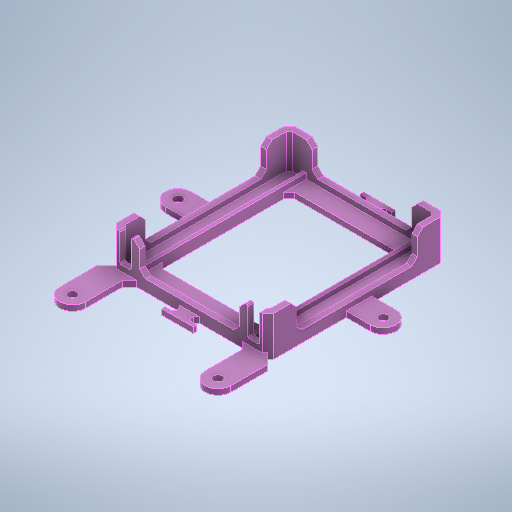
# Autodesk Inventor part: Battery-Holder-SPG27-1x4-A
Saved by Autodesk Inventor 2025.3 (Build 293356000, 356)
## iProperties
Created: 2025-09-09
Part Number: Battery-Holder-SPG27-1x4-A
Material: 一般
Document SubType Name: Modeling
Designer: daisuke
Density: 1 g/cm^3
Appearance: 滑らか - 紫
Author: daisuke
Autodesk Inventor part; units mm, degrees
ref_plane "YZ Plane" through (0, 0, 0) normal (1, 0, 0) x (0, 1, 0)
ref_plane "XZ Plane" through (0, 0, 0) normal (0, 1, 0) x (-1, 0, 0)
ref_plane "XY Plane" through (0, 0, 0) normal (0, 0, 1) x (1, 0, 0)
sketch "スケッチ1" plane through (0, 0, 0) normal (0, 0, 1) x (1, 0, 0)
  line L0 (-35.3559, -10) -> (35.3559, -10) construction
  line L1 (0, 64.852) -> (0, -64.852) construction
  circle A0 centre (-25.5, -27.5) radius 4.5
  circle A1 centre (25.5, -27.5) radius 4.5
  circle A2 centre (36, 20) radius 4.5
  circle A3 centre (-36, 20) radius 4.5
  line L2 (-25.5, 48.5) -> (25.5, 48.5)
  line L3 (25.5, 48.5) -> (25.5, -10)
  line L4 (25.5, -10) -> (-25.5, -10)
  line L5 (-25.5, -10) -> (-25.5, 48.5)
  line L6 (-27.5, 50.5) -> (27.5, 50.5)
  line L7 (27.5, 50.5) -> (27.5, -12)
  line L8 (27.5, -12) -> (-27.5, -12)
  line L9 (-27.5, -12) -> (-27.5, 50.5)
  line L10 (-27.5, 24.5) -> (-36, 24.5)
  line L11 (-36, 15.5) -> (-27.5, 15.5)
  line L12 (27.5, 24.5) -> (36, 24.5)
  line L13 (36, 15.5) -> (27.5, 15.5)
  line L14 (-21, -12) -> (-21, -27.5)
  line L15 (21, -27.5) -> (21, -12)
  line L16 (-30, -27.5) -> (-30, -14.5)
  line L17 (-30, -14.5) -> (-27.5, -12)
  line L18 (27.5, -12) -> (30, -14.5)
  line L19 (30, -14.5) -> (30, -27.5)
  line L20 (-19.5, 42.5) -> (19.5, 42.5)
  line L21 (19.5, 42.5) -> (19.5, -4)
  line L22 (19.5, -4) -> (-19.5, -4)
  line L23 (-19.5, -4) -> (-19.5, 42.5)
  circle A4 centre (-25.5, -27.5) radius 1.6
  circle A5 centre (25.5, -27.5) radius 1.6
  circle A6 centre (36, 20) radius 1.6
  circle A7 centre (-36, 20) radius 1.6
  line L24 (-21, -14.5) -> (-18.5, -12)
  line L25 (21, -14.5) -> (18.5, -12)
  line L26 (-2.5, -12) -> (-2.5, -15)
  line L27 (-2.5, -15) -> (-5.5, -15)
  line L28 (-5.5, -15) -> (-5.5, -16.2)
  line L29 (-5.5, -16.2) -> (5.5, -16.2)
  line L30 (5.5, -16.2) -> (5.5, -15)
  line L31 (5.5, -15) -> (2.5, -15)
  line L32 (2.5, -15) -> (2.5, -12)
  line L33 (-2.5, 50.5) -> (-2.5, 53.5)
  line L34 (-2.5, 53.5) -> (-5.5, 53.5)
  line L35 (-5.5, 53.5) -> (-5.5, 54.7)
  line L36 (-5.5, 54.7) -> (5.5, 54.7)
  line L37 (5.5, 54.7) -> (5.5, 53.5)
  line L38 (5.5, 53.5) -> (2.5, 53.5)
  line L39 (2.5, 53.5) -> (2.5, 50.5)
  line L40 (-20.7, 48.5) -> (-19.5, 48.5)
  line L41 (-19.5, 48.5) -> (-19.5, -10)
  line L42 (-19.5, -10) -> (-20.7, -10)
  line L43 (-20.7, -10) -> (-20.7, 48.5)
  line L44 (20.7, 48.5) -> (19.5, 48.5)
  line L45 (19.5, 48.5) -> (19.5, -10)
  line L46 (19.5, -10) -> (20.7, -10)
  line L47 (20.7, -10) -> (20.7, 48.5)
  point P0 (0, 0)
  point P1 (0, 0)
  point P2 (0, -10)
  point P3 (-25.5, 7.5)
  point P4 (25.5, 7.5)
  point P5 (-36, 43)
  point P6 (36, 43)
  point P7 (0, -10)
  point P8 (0, 50.5)
  point P9 (27.5, 19.25)
  point P10 (25.5, 19.25)
  point P11 (0, 42.5)
  point P12 (19.5, 19.25)
  dimension "d0" = 10
  dimension "d1" = 35
  dimension "d2" = 51
  dimension "d3" = 23
  dimension "d4" = 43
  dimension "d5" = 72
  dimension "d6" = 9
  dimension "BAT_W" = 51
  dimension "BAT_L" = 58.5
  dimension "d9" = 2
  dimension "d10" = 2
  dimension "d11" = 135
  dimension "d12" = 135
  dimension "d13" = 6
  dimension "d14" = 6
  dimension "d15" = 3.2
  dimension "d27" = 3
  dimension "d28" = 3
  dimension "d29" = 1.2
  dimension "d30" = 5
  dimension "d36" = 1.2
  dimension "d37" = 1.2
  constraints: 96 end point, 26 point on line, 19 perpendicular, 12 parallel, 9 coincident, 9 horizontal, 8 centre point, 8 midpoint, 8 point on circle, 8 tangent, 7 horizontal alignment, 6 collinear, 6 equal radius, 4 vertical, 3 equal length, 3 symmetric about line, 3 vertical alignment, 2 other
  measures "d0" distance from line of point (0, 0) L0
  measures "d1" distance of point (25.5, -27.5) point (25.5, 7.5)
  measures "d2" distance of point (-25.5, -27.5) point (25.5, -27.5)
  measures "d3" distance of point (-36, 20) point (-36, 43)
  measures "d4" vertical distance of point (0, 0) point (36, 43)
  measures "d5" distance of point (36, 43) point (-36, 43)
  measures "d6" diameter of A0
  measures "BAT_W" distance of L3.end L4.end
  measures "BAT_L" distance of L2.end L3.end
  measures "d9" distance between parallel lines of L6 L2
  measures "d10" distance between parallel lines of L7 L3
  measures "d11" angle of L9 L17
  measures "d12" angle of L7 L18
  measures "d13" distance between parallel lines of L2 L20
  measures "d14" distance between parallel lines of L3 L21
  measures "d15" diameter of A4
  measures "d27" distance of L26.start L26.end
  measures "d28" distance of L26.end L27.end
  measures "d29" distance of L27.end L28.end
  measures "d30" distance between parallel lines of L32 L26
  measures "d36" distance of L41.end L42.end
  measures "d37" distance between parallel lines of L47 L45
extrude "ベース" add sketch "スケッチ1" along normal blind 2 contours A0 | A0 L16 L17 L8 L14 | L14 L8 L24 | L8 L9 L6 L7 | L11 A3 L10 L9 | A3 | L8 L15 L25 | L8 L18 L19 A1 L15 | A1 | L7 L12 A2 L13 | A2 | L2 L43 L4 L5 | L2 L41 L23 L4 L43 | L2 L45 L20 L41 | L2 L47 L4 L45 L21 | L41 L22 L45 L4 | L2 L3 L4 L47
extrude "壁" add sketch "スケッチ1" along normal blind 14 contours L8 L9 L6 L7
sketch "スケッチ4" plane through (0, 0, 14) normal (0, 0, 1) x (1, 0, 0)
  line L0 (-27.5, 15.5) -> (-27.5, -12) projected
  line L1 (-25.5, 48.5) -> (-25.5, -10) projected
  line L2 (-27.5, -2) -> (-25.5, -2)
  line L3 (-25.5, -2) -> (-25.5, 40.5)
  line L4 (-25.5, 40.5) -> (-27.5, 40.5)
  line L5 (-27.5, 40.5) -> (-27.5, -2)
  line L6 (27.5, 50.5) -> (-27.5, 50.5) projected
  line L7 (-17.5, 48.5) -> (17.5, 48.5)
  line L8 (17.5, 48.5) -> (17.5, 50.5)
  line L9 (17.5, 50.5) -> (-17.5, 50.5)
  line L10 (-17.5, 50.5) -> (-17.5, 48.5)
  line L11 (-27.5, 50.5) -> (-27.5, -12) projected
  line L12 (-25.5, 48.5) -> (25.5, 48.5) projected
  line L13 (-18.5, -12) -> (18.5, -12) projected
  line L14 (-17.5, -12) -> (17.5, -12)
  line L15 (17.5, -12) -> (17.5, -10)
  line L16 (17.5, -10) -> (-17.5, -10)
  line L17 (-17.5, -10) -> (-17.5, -12)
  line L18 (25.5, -10) -> (25.5, 48.5) projected
  line L19 (27.5, 24.5) -> (27.5, 50.5) projected
  line L20 (25.5, -2) -> (27.5, -2)
  line L21 (27.5, -2) -> (27.5, 40.5)
  line L22 (27.5, 40.5) -> (25.5, 40.5)
  line L23 (25.5, 40.5) -> (25.5, -2)
  line L24 (25.5, -10) -> (-25.5, -10) projected
  point P0 (0, 0)
  point P1 (-25.5, 19.25)
  point P2 (0, 48.5)
  dimension "d23" = 10
  dimension "d24" = 10
  constraints: 32 end point, 8 parallel, 6 point on line, 5 collinear, 4 horizontal, 4 midpoint, 4 perpendicular
  measures "d23" distance between parallel lines of L6 L4
  measures "d24" distance between parallel lines of L11 L10
extrude "壁切り欠き" cut sketch "スケッチ4" against normal blind 10 contours L5 L4 L1 L2 L0 | L6 L8 L7 L10 | L16 L15 L13 L17 | L19 L21 L20 L18 L22
extrude "押し出し4" add sketch "スケッチ1" along normal blind 2 contours L8 L32 L31 L30 L29 L28 L27 L26 | L33 L34 L35 L36 L37 L38 L39 L6
extrude "押し出し5" add sketch "スケッチ1" along normal blind 4 contours L2 L41 L23 L4 L43 | L2 L47 L4 L45 L21
chamfer "面取り1" distance 2 angle 45 4 edges at (-19.5, 42.5, 1) (19.5, 42.5, 1) (-19.5, -4, 1) (19.5, -4, 1)
chamfer "面取り2" distance 2 angle 45 16 edges at (-26.5, -2, 14) (-17.5, -11, 14) (-17.5, -11, 4) (17.5, -11, 4) (17.5, -11, 14) (-26.5, 40.5, 14) (-26.5, 40.5, 4) (-17.5, 49.5, 14) (-17.5, 49.5, 4) (26.5, -2, 14) (26.5, -2, 4) (26.5, 40.5, 14) (26.5, 40.5, 4) (17.5, 49.5, 14) (17.5, 49.5, 4) (-26.5, -2, 4)
chamfer "面取り3" distance 1 angle 45 4 edges at (-25.5, -10, 8) (25.5, -10, 8) (-25.5, 48.5, 8) (25.5, 48.5, 8)
chamfer "面取り4" distance 2 angle 45 4 edges at (-27.5, -12, 8) (27.5, -12, 8) (27.5, 50.5, 7) (-27.5, 50.5, 7)
sketch "スケッチ5" plane through (0, 0, 14) normal (0, 0, 1) x (1, 0, 0)
  line L0 (24.5, -10) -> (19.5, -10) projected
  line L1 (25.5, -12) -> (18.5, -12) projected
  line L2 (24.5, -10) -> (20.5, -10)
  line L3 (20.5, -10) -> (20.5, -12)
  line L4 (20.5, -12) -> (24.5, -12)
  line L5 (24.5, -12) -> (24.5, -10)
  line L6 (-24.5, -10) -> (-20.5, -10)
  line L7 (-20.5, -10) -> (-20.5, -12)
  line L8 (-20.5, -12) -> (-24.5, -12)
  line L9 (-24.5, -12) -> (-24.5, -10)
  point P0 (0, 0)
  dimension "d52" = 4
  dimension "d53" = 4
  constraints: 16 end point, 4 parallel, 3 point on line, 2 horizontal, 2 perpendicular, 1 coincident
  measures "d52" distance of L4.end L3.end
  measures "d53" distance between parallel lines of L7 L9
extrude "押し出し6" cut sketch "スケッチ5" against normal up to surface (10 mm away)
chamfer "面取り5" distance 0.4 angle 45 8 edges at (24.5, -11, 14) (24.5, -11, 4) (20.5, -11, 4) (20.5, -11, 14) (-24.5, -11, 14) (-20.5, -11, 14) (-24.5, -11, 4) (-20.5, -11, 4)
chamfer "面取り6" distance 1 angle 45 8 edges at (2.5, -12, 1) (2.5, -15, 1) (-2.5, -12, 1) (-2.5, -15, 1) (2.5, 50.5, 1) (2.5, 53.5, 1) (-2.5, 50.5, 1) (-2.5, 53.5, 1)
equation "\"d10\" = d9"
equation "\"d12\" = d11"
equation "\"d14\" = d13"
equation "\"d37\" = d36"
equation "\"d24\" = d23"
equation "\"d53\" = d52"
